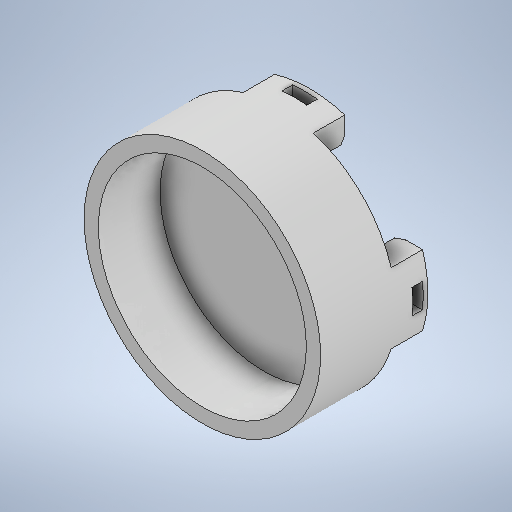
# Autodesk Inventor part: Module_Base
Saved by Autodesk Inventor 2025.1 (Build 291241020, 241B)
## iProperties
Created: 2024-10-12
Part Number: Module_Base
Material: 일반
Document SubType Name: Modeling
Designer: SEON06
Density: 1 g/cm^3
Appearance: 기본값
Author: SEON06
## iProperties of the stored document Module_Base_3D 인쇄.ipt
Created: 2024-10-12
Part Number: Module_Base_3D 인쇄
Material: 일반
Document SubType Name: Modeling
Designer: SEON06
Density: 1 g/cm^3
Appearance: 기본값
Author: SEON06
Autodesk Inventor part; units mm, degrees
ref_plane "YZ Plane" through (0, 0, 0) normal (1, 0, 0) x (0, 1, 0)
ref_plane "XY Plane" through (0, 0, 0) normal (0, 0, 1) x (1, 0, 0)
sketch "스케치1" plane through (0, 0, 0) normal (0, 0, 1) x (1, 0, 0)
  circle A0 centre (0, 0) radius 24.9
  circle A1 centre (0, 0) radius 20.1
  line L0 (-7.4, 24.9) -> (-7.4, 18.6882)
  line L1 (-7.4, 24.9) -> (7.4, 24.9)
  line L2 (7.4, 24.9) -> (7.4, 18.6882)
  line L3 (-24.9, -7.4) -> (-18.6882, -7.4)
  line L4 (-24.9, 7.4) -> (-18.6882, 7.4)
  line L5 (7.4, -24.9) -> (7.4, -18.6882)
  line L6 (-7.4, -24.9) -> (-7.4, -18.6882)
  line L7 (24.9, 7.4) -> (18.6882, 7.4)
  line L8 (24.9, -7.4) -> (18.6882, -7.4)
  circle A2 centre (0, 0) radius 21.9
  point P0 (0, 24.9)
  point P1 (-7.4, -23.775)
  point P2 (7.4, -23.775)
  point P3 (-23.775, 7.4)
  point P4 (-23.775, -7.4)
  point P5 (7.4, 23.775)
  point P6 (-7.4, 23.775)
  point P7 (18.6882, -7.4)
  point P8 (23.775, -7.4)
  point P9 (23.775, 7.4)
  dimension "d0" = 49.8
  dimension "d1" = 4.8
  dimension "d2" = 14.8
  dimension "d5" = 360
  dimension "d22" = 3
  constraints: 18 end point, 3 centre point, 2 point on circle, 1 coincident, 1 horizontal, 1 midpoint, 1 perpendicular, 1 tangent, 1 vertical, 1 vertical alignment, 25 other
  measures "d0" diameter of A0
  measures "d1" radial gap between concentric circles of A0 A1
  measures "d2" distance of L0.start L1.end
  measures "d22" radial gap between concentric circles of A0 A2
extrude "돌출1" add sketch "스케치1" along normal blind 16 contours A0 L8 A2 L7 | L7 A2 L2 A0 | A0 L5 A2 L8 | L2 A2 L0 A0 | A0 L6 A2 L5 | A0 L3 A2 L6 | L0 A2 L4 A0 | A0 L4 A2 L3
extrude "돌출2" add sketch "스케치1" along normal blind 3 contours A2 L8 A1 L7 | L7 A1 L2 A2 | A2 L5 A1 L8 | L2 A1 L0 A2 | A1 | A2 L6 A1 L5 | L0 A1 L4 A2 | A2 L3 A1 L6 | L4 A1 L3 A2
extrude "돌출3" add sketch "스케치1" against normal blind 6.6 contours A0 L8 A2 L7 | L2 A2 L0 A0 | A2 L8 A1 L7 | A0 L6 A2 L5 | L2 A1 L0 A2 | A2 L6 A1 L5 | A0 L4 A2 L3 | L4 A1 L3 A2
ref_plane "작업 평면1" through (0, -24.9, 0) normal (0, 1, 0) x (-1, 0, 0)
sketch "스케치2" plane through (0, -24.9, 0) normal (0, 1, 0) x (-1, 0, 0)
  line L0 (-7.4, 0) -> (7.4, 0) projected
  line L1 (-7.4, 0) -> (-7.4, -6.6) projected
  line L2 (-7.4, -3.4) -> (3.75, -3.4)
  line L3 (24.9, 16) -> (-24.9, 16) projected
  line L4 (-23.775, 0) -> (-7.4, 0) projected
  line L5 (-7.4, 0) -> (-7.4, -6.6) projected
  line L6 (7.4, -6.6) -> (-7.4, -6.6) projected
  line L7 (7.4, 0) -> (7.4, -6.6) projected
  line L8 (7.4, 0) -> (23.775, 0) projected
  line L9 (23.775, 0) -> (23.775, -6.6) projected
  line L10 (23.775, -6.6) -> (23.775, -6.6) projected
  line L11 (23.775, 0) -> (23.775, -6.6) projected
  line L12 (23.775, 0) -> (7.4, 0) projected
  line L13 (7.4, 0) -> (7.4, -6.6) projected
  line L14 (-7.4, -6.6) -> (7.4, -6.6) projected
  line L15 (-7.4, 0) -> (-7.4, -6.6) projected
  line L16 (-7.4, 0) -> (-23.775, 0) projected
  line L17 (-23.775, 0) -> (-23.775, -6.6) projected
  line L18 (-23.775, -6.6) -> (-23.775, -6.6) projected
  line L19 (-23.775, 0) -> (-23.775, -6.6) projected
  line L20 (-7.4, -5.6) -> (7.4, -5.6)
  line L21 (-2.6, -5.6) -> (-2.6, -3.4)
  line L22 (2.6, -5.6) -> (2.6, -3.4)
  point P0 (0, 0)
  point P1 (0, 0)
  dimension "d13" = 3.4
  dimension "d14" = 2.2
  dimension "d15" = 5.2
  dimension "d16" = 2.6
  constraints: 8 end point, 7 point on line, 3 perpendicular, 1 horizontal, 1 midpoint
  measures "d13" distance between parallel lines of L0 L2
  measures "d14" distance between parallel lines of L2 L20
  measures "d15" distance between parallel lines of L21 L22
  measures "d16" distance from line of point (0, 0) L22
extrude "돌출4" cut sketch "스케치2" along normal through all contours L2 L22 L20 L21
pattern_circular "원형 패턴1" count 2 over 90 about axis through (0, 0, 0) along (0, 0, 1) of "돌출4"
chamfer "모따기1" distance 0.5 angle 45 16 edges at (0, 20.1, -3.4) (-2.6, 19.9311, -4.5) (0, 20.1, -5.6) (2.6, 19.9311, -4.5) (20.1, 0, -3.4) (19.9311, 2.6, -4.5) (20.1, 0, -5.6) (19.9311, -2.6, -4.5) (2.6, -19.9311, -4.5) (0, -20.1, -3.4) (-2.6, -19.9311, -4.5) (0, -20.1, -5.6) (-20.1, 0, -3.4) (-19.9311, 2.6, -4.5) (-20.1, 0, -5.6) (-19.9311, -2.6, -4.5)
chamfer "모따기2" distance 0.8 angle 60 1 edges at (0, 20.1, -6.6) measured on face at (0, 20.1, -6.5)
chamfer "모따기3" distance 0.8 angle 60 1 edges at (20.1, 0, -6.6) measured on face at (20.1, 0, -6.5)
chamfer "모따기4" distance 0.8 angle 60 1 edges at (-20.1, 0, -6.6) measured on face at (-20.1, 0, -6.5)
chamfer "모따기5" distance 0.8 angle 60 1 edges at (0, -20.1, -6.6) measured on face at (0, -20.1, -6.5)
equation "\"d16\" = 0.5 * d15"
